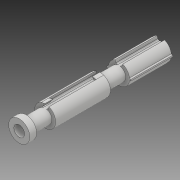
# Autodesk Inventor part: 2101_Rx Coil Body_V2
Saved by Autodesk Inventor 2020 (Build 240168000, 168)
## iProperties
Created: 2019-06-18
Part Number: 2101_Rx Coil Body_V2
Material: Generic
Document SubType Name: Modeling
Designer: RFLab
Density: 1 g/cm^3
Appearance: Default
Author: RFLab
Autodesk Inventor part; units mm, degrees
ref_plane "YZ Plane" through (0, 0, 0) normal (1, 0, 0) x (0, 1, 0)
ref_plane "XZ Plane" through (0, 0, 0) normal (0, 1, 0) x (-1, 0, 0)
ref_plane "XY Plane" through (0, 0, 0) normal (0, 0, 1) x (1, 0, 0)
sketch "Sketch1" plane through (0, 0, 0) normal (0, 1, 0) x (-1, 0, 0)
  circle A0 centre (0, 0) radius 3.5
  circle A1 centre (0, 0) radius 4.5
  dimension "OD" = 9
  dimension "ID" = 7
  constraints: 2 centre point, 2 coincident
  measures "OD" diameter of A1
  measures "ID" diameter of A0
extrude "Extrusion1" add sketch "Sketch1" along normal blind 12
ref_plane "Work Plane1" through (0, 0, -10) normal (-1, 0, 0) x (0, 0, 1)
sketch "Sketch2" plane through (0, 0, -10) normal (-1, 0, 0) x (0, 0, 1)
  circle A0 centre (14.67, 11.4) radius 0.6
  line L0 (5.5, 0) -> (14.5, 0) projected
  line L1 (14.5, 0) -> (14.5, 12) projected
  point P0 (10, 0)
  point P1 (14.5, 11.9754)
  dimension "d10" = 1.2
  dimension "d12" = 0.17
  dimension "d119" = 0.6
  constraints: 1 coincident, 1 point on line, 3 other
  measures "d12" horizontal distance of point (14.5, 0) point (14.67, 11.4)
  measures "d119" vertical distance of L1.end point (14.67, 11.4)
sketch "Sketch3" plane through (0, 0, 0) normal (0, -1, 0) x (1, 0, 0)
  circle A0 centre (0, 0) radius 3.5
  circle A1 centre (0, 0) radius 6.95
  dimension "d21" = 7
  dimension "OOD" = 13.9
  constraints: 2 centre point, 2 coincident
  measures "d21" diameter of A0
  measures "OOD" diameter of A1
extrude "Extrusion2" add sketch "Sketch3" along normal blind 36
sketch "Sketch4" plane through (0, -36, 0) normal (0, -1, 0) x (1, 0, 0)
  circle A0 centre (0, 0) radius 3.5
  circle A1 centre (0, 0) radius 4.5
  dimension "d25" = 7
  dimension "d26" = 9
  constraints: 2 centre point, 2 coincident
  measures "d25" diameter of A0
  measures "d26" diameter of A1
extrude "Extrusion3" add sketch "Sketch4" along normal blind 12
sketch "Sketch5" plane through (0, 0, -10) normal (-1, 0, 0) x (0, 0, 1)
  circle A0 centre (14.67, -36.6) radius 0.6
  line L0 (14.5, -36) -> (14.5, -48) projected
  line L1 (3.05, -36) -> (16.95, -36) projected
  point P0 (10, 0)
  point P1 (14.5, -37.1754)
  point P2 (14.5, -36.0246)
  dimension "d29" = 1.2
  dimension "d30" = 0.17
  dimension "d31" = 0.6
  constraints: 2 point on circle, 2 point on line, 1 centre point
  measures "d29" diameter of A0
  measures "d30" horizontal distance of A0.end A0.centre
  measures "d31" distance from line of L1 A0.centre
sketch "Sketch6" plane through (0, 0, 0) normal (0, 1, 0) x (1, 0, 0)
  arc A0 (-2, -4.0311) -> (2, -4.0311) centre (0, 0) ccw
  arc A1 (-2.5, -6.4848) -> (2.5, -6.4848) centre (0, 0) ccw
  circle A2 centre (0, 0) radius 6.95 projected
  line L0 (2.5, -6.4848) -> (2, -4.0311)
  circle A3 centre (0, 0) radius 4.5 projected
  line L1 (-2, -4.0311) -> (-2.5, -6.4848)
  line L2 (0, -9.73) -> (0, 9.73) projected
  dimension "d42" = 5
  dimension "d43" = 4
  dimension "d45" = 2
  dimension "d46" = 2.5
  constraints: 6 point on circle, 4 end point, 2 centre point, 2 coincident, 2 other
  measures "d42" distance of L1.end L0.start
  measures "d43" distance of L1.start L0.end
  measures "d45" distance from line of L0.end L2
  measures "d46" distance from line of L0.start L2
extrude "Extrusion4" cut sketch "Sketch6" against normal blind 121.2 contours A0 L2 A1 L1 | A0 L0 A1 L2
fillet "Fillet1" radius 1 2 edges at (2, -18, 4.0311) (-2, -18, 4.0311)
ref_plane "Work Plane5" through (-10, 45, 0) normal (0, -1, 0) x (1, 0, 0)
ref_plane "Work Plane4" through (-10, 0, 0) normal (0, -1, 0) x (1, 0, 0)
sketch "Sketch13" plane through (0, 12, 0) normal (0, 1, 0) x (1, 0, 0)
  circle A0 centre (0, 0) radius 3.5
  circle A1 centre (0, 0) radius 6.95
  dimension "d75" = 13.9
  dimension "d105" = 7
  constraints: 2 centre point, 2 coincident
  measures "d75" diameter of A1
  measures "d105" diameter of A0
extrude "Extrusion9" add sketch "Sketch13" along normal blind 28
sketch "Sketch17" plane through (2.5, -36, 6.4848) normal (-0.9798625, 0, 0.1996736) x (0.1996736, 0, 0.9798625)
  line L0 (-1.3556, 36) -> (0, 36) projected
  line L1 (0, 36) -> (-2, 36)
  line L2 (-2, 36) -> (-2, 31)
  line L3 (-2, 31) -> (0, 31)
  line L4 (0, 31) -> (0, 36)
  point P0 (-6.8534, 36)
  point P1 (-6.5156, 60)
  dimension "d94" = 2
  dimension "d95" = 5
  constraints: 8 end point, 2 parallel, 1 horizontal, 1 perpendicular, 1 other
  measures "d94" distance of L3.end L2.end
  measures "d95" distance between parallel lines of L3 L1
extrude "Extrusion13" add sketch "Sketch17" along normal blind 2.5
sketch "Sketch18" plane through (-2.5, -36, 6.4848) normal (0.9798625, 0, 0.1996736) x (0.1996736, 0, -0.9798625)
  line L0 (0, 0) -> (0, 36) projected
  line L1 (0, 0) -> (2, 0)
  line L2 (2, 0) -> (2, 5)
  line L3 (2, 5) -> (0, 5)
  line L4 (0, 5) -> (0, 0)
  point P0 (6.8534, 36)
  dimension "d98" = 2
  dimension "d99" = 5
  constraints: 8 end point, 2 parallel, 1 horizontal, 1 perpendicular
  measures "d98" distance of L3.end L2.end
  measures "d99" distance of L3.end L0.start
extrude "Extrusion14" add sketch "Sketch18" along normal blind 2.5
sketch "Sketch20" plane through (0, 40, 0) normal (0, 1, 0) x (1, 0, 0)
  circle A0 centre (0, 0) radius 3.5 construction
  circle A1 centre (0, 0) radius 6.95 construction
  arc A2 (2.5, -6.4848) -> (-2.5, -6.4848) centre (0, 0) ccw projected
  circle A3 centre (0, 0) radius 4.5
  arc A4 (-2.5, -6.4848) -> (2.5, -6.4848) centre (0, 0) ccw
  arc A5 (2.5, -6.4848) -> (-2.5, -6.4848) centre (0, 0) ccw projected
  line L0 (2.5, -6.4848) -> (0, 0)
  line L1 (0, 0) -> (-2.5, -6.4848)
  point P0 (0, -4.5)
  point P1 (1.6187, -4.1988)
  point P2 (-1.6187, -4.1988)
  constraints: 4 end point, 2 point on circle, 1 centre point, 1 coincident, 1 concentric, 3 other
extrude "Extrusion16" cut sketch "Sketch20" against normal up to surface (28 mm away) contours A4 L1 A3 L0
fillet "Fillet3" radius 1 2 edges at (1.6187, 26, 4.1988) (-1.6187, 26, 4.1988)
sketch "Sketch21" plane through (0, -48, 0) normal (0, -1, 0) x (1, 0, 0)
  circle A0 centre (0, 0) radius 3.5 projected
  circle A1 centre (0, 0) radius 6.95
  dimension "d109" = 13.9
  constraints: 1 centre point, 1 coincident
  measures "d109" diameter of A1
extrude "Extrusion17" add sketch "Sketch21" along normal blind 5
sketch "Sketch22" plane through (0, -48, 0) normal (0, 1, 0) x (1, 0, 0)
  circle A0 centre (0, 0) radius 6.95 projected
  circle A1 centre (0, 0) radius 4.5 projected
extrude "Extrusion18" cut sketch "Sketch22" against normal blind 0.5
sketch "Sketch23" plane through (0, 12, 0) normal (0, -1, 0) x (1, 0, 0)
  arc A0 (-0.8283, 4.4231) -> (0.8283, 4.4231) centre (0, 0) ccw projected
  arc A1 (-1.9454, 5.0463) -> (-0.8283, 4.4231) centre (-1.0124, 5.406) ccw projected
  line L0 (-1.9454, 5.0463) -> (-2.5, 6.4848) projected
  arc A2 (-2.5, 6.4848) -> (2.5, 6.4848) centre (0, 0) ccw projected
  line L1 (2.5, 6.4848) -> (1.9454, 5.0463) projected
  arc A3 (0.8283, 4.4231) -> (1.9454, 5.0463) centre (1.0124, 5.406) ccw projected
extrude "Extrusion19" cut sketch "Sketch23" against normal blind 0.5
chamfer "Chamfer1" distance 2 angle 45 2 edges at (-0.349, -2.5, 5.0242) (0.349, -33.5, 5.0242)
ref_plane "Work Plane6" through (0, -18, 0) normal (0, 1, 0) x (1, 0, 0)
sketch "Sketch24" plane through (0, 40, 0) normal (0, 1, 0) x (1, 0, 0)
  line L0 (7.85, -0.45) -> (7.85, 0.45)
  line L1 (7.85, 0.45) -> (6.9045, 0.7941)
  arc A0 (2.5, -6.4848) -> (-2.5, -6.4848) centre (0, 0) ccw projected
  line L2 (7.85, -0.45) -> (6.9045, -0.7941)
  line L3 (-7.85, -0.45) -> (-7.85, 0.45)
  line L4 (-7.85, 0.45) -> (-6.9045, 0.7941)
  arc A1 (2.5, -6.4848) -> (-2.5, -6.4848) centre (0, 0) ccw projected
  line L5 (-7.85, -0.45) -> (-6.9045, -0.7941)
  dimension "d121" = 0.9
  dimension "d123" = 0.9
  dimension "d125" = 110
  dimension "d126" = 110
  dimension "d128" = 0.9
  dimension "d129" = 0.9
  dimension "d130" = 110
  dimension "d131" = 110
  constraints: 12 end point, 4 point on circle, 2 equal length, 2 vertical
  measures "d121" distance of L0.start L0.end
  measures "d123" distance edge to line of A0 L0
  measures "d125" angle of L2 L0
  measures "d126" angle of L0 L1
  measures "d128" distance of L3.start L3.end
  measures "d129" distance edge to line of A0 L3
  measures "d130" angle of L3 L4
  measures "d131" angle of L3 L5
extrude "Extrusion20" add sketch "Sketch24" against normal up to surface (27.5 mm away)
equation "\"d21\" = ID"
equation "\"d25\" = ID"
equation "\"d26\" = OD"
equation "\"d75\" = OOD"
equation "\"d105\" = ID"
equation "\"d109\" = OOD"
body "Solid1"
